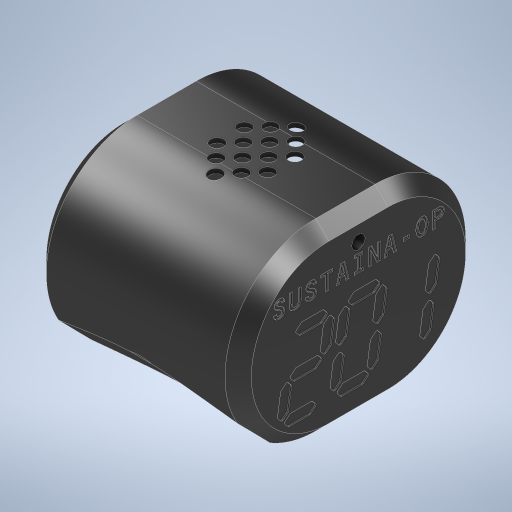
# Autodesk Inventor part: HeadCover
Saved by Autodesk Inventor 2024.2 (Build 282272000, 272)
## iProperties
Created: 2024-06-13
Part Number: HeadCover
Material: ABS Plastic
Document SubType Name: Modeling
Designer: Masato Kubotera
Density: 1.06 g/cm^3
Appearance: Glossy - Black
Author: Masato Kubotera
Autodesk Inventor part; units mm, degrees
(part 1 of 2)
ref_plane "YZ Plane" through (0, 0, 0) normal (1, 0, 0) x (0, 1, 0)
ref_plane "XZ Plane" through (0, 0, 0) normal (0, 1, 0) x (-1, 0, 0)
ref_plane "XY Plane" through (0, 0, 0) normal (0, 0, 1) x (1, 0, 0)
derived "HeadSideFrame_.ipt"
sketch "Sketch1" plane through (0, 0, 0) normal (0, 1, 0) x (-1, 0, 0)
  line L0 (-16.25, -1.5) -> (16.25, -1.5)
  line L1 (-7.25, -1.5) -> (-7.25, 3.5) construction
  line L2 (-7.25, 3.5) -> (7.25, 3.5) construction
  line L3 (0, 3.5) -> (0, -1.5) construction
  line L4 (7.25, -1.5) -> (7.25, 3.5) construction
  line L5 (-13.25, 1) -> (13.25, 1) construction
  line L6 (-7.3, -1.5) -> (-7.3, 3.5)
  line L7 (-7.3, 3.5) -> (7.3, 3.5)
  arc A0 (-4.3, 3.5) -> (-7.3, 3.5) centre (-5.8, 3.5) ccw
  arc A1 (7.3, 3.5) -> (4.3, 3.5) centre (5.8, 3.5) ccw
  line L8 (7.3, -1.5) -> (7.3, 3.5)
  line L9 (-16.25, -1.5) -> (-16.25, 32)
  line L10 (16.25, -1.5) -> (16.25, 65)
  ellipse E0 centre (-16.25, 65) end of major axis (18.25, 65) minor radius 35 (-16.25, 30) -> (-16.25, 100) ccw construction
  line L11 (-16.25, 30) -> (-16.25, 100) construction
  line L12 (-16.25, 65) -> (18.25, 65) construction
  ellipse E1 centre (-16.25, 65) end of major axis (16.25, 65) minor radius 33 (-16.25, 32) -> (16.25, 65) ccw construction
  line L13 (-16.25, 32) -> (-38.75, 32)
  line L14 (-16.25, 98) -> (-38.75, 98)
  line L15 (-27.5, 98) -> (-27.5, 32) construction
  ellipse E2 centre (-38.75, 65) end of major axis (-71.25, 65) minor radius 33 (-38.75, 98) -> (-71.1715, 67.2921) ccw
  ellipse E3 centre (-38.75, 65) end of major axis (-73.25, 65) minor radius 35 (-38.75, 100) -> (-38.75, 30) ccw construction
  line L16 (-38.75, 30) -> (-16.25, 30) construction
  line L17 (-38.75, 100) -> (-16.25, 100) construction
  line L18 (-10.25, 30) -> (10.25, 30)
  line L19 (12.25, 28) -> (12.25, 11)
  line L20 (10.25, 9) -> (-10.25, 9)
  line L21 (-12.25, 11) -> (-12.25, 28)
  line L22 (-12.25, 30) -> (12.25, 9) construction
  line L23 (12.25, 30) -> (-12.25, 9) construction
  arc A2 (-10.25, 30) -> (-12.25, 28) centre (-10.25, 28) ccw
  arc A3 (-12.25, 11) -> (-10.25, 9) centre (-10.25, 11) ccw
  arc A4 (10.25, 9) -> (12.25, 11) centre (10.25, 11) ccw
  arc A5 (12.25, 28) -> (10.25, 30) centre (10.25, 28) ccw
  line L24 (-38.75, 30) -> (-38.75, 100) construction
  line L25 (-38.75, 32) -> (-38.75, 34.8706)
  line L26 (-38.75, 34.8706) -> (-71.1715, 67.2921)
  line L27 (-62.0208, 45.9792) -> (-108, 0) construction
  line L28 (-108, 0) -> (0, 0) construction
  ellipse E4 centre (-38.75, 65) end of major axis (-71.25, 65) minor radius 33 (-71.1715, 67.2921) -> (-38.75, 32) ccw construction
  ellipse E5 centre (-16.25, 65) end of major axis (16.25, 65) minor radius 33 (16.25, 65) -> (-16.25, 98) ccw
  line L29 (-55, 91.5815) -> (0, 91.5815) construction
  line L30 (0, 91.5815) -> (0, 86.5815) construction
  line L31 (0, 86.5815) -> (-55, 86.5815) construction
  line L32 (-55, 86.5815) -> (-55, 91.5815) construction
  line L33 (-55, 91.5815) -> (0, 86.5815) construction
  line L34 (0, 91.5815) -> (-55, 86.5815) construction
  line L35 (-47.5, 91.5815) -> (-47.5, 96.7815) construction
  line L36 (-47.5, 96.7815) -> (-7.5, 96.7815) construction
  line L37 (-7.5, 96.7815) -> (-7.5, 91.5815) construction
  line L38 (-46, 91.5815) -> (-46, 86.5815) construction
  line L39 (-52, 89.0815) -> (-3, 89.0815) construction
  line L40 (-9, 91.5815) -> (-9, 86.5815) construction
  line L41 (-8.95, 86.5315) -> (-46.05, 86.5315)
  line L42 (-46.05, 86.5315) -> (-46.05, 91.6315)
  line L43 (-46.05, 91.6315) -> (-8.95, 91.6315)
  line L44 (-8.95, 91.6315) -> (-8.95, 86.5315)
  line L45 (-8.95, 86.5315) -> (-46.05, 91.6315) construction
  line L46 (-46.05, 86.5315) -> (-8.95, 91.6315) construction
  arc A6 (-43.05, 91.6315) -> (-46.05, 91.6315) centre (-44.55, 91.6315) ccw
  arc A7 (-46.05, 86.5315) -> (-43.05, 86.5315) centre (-44.55, 86.5315) ccw
  arc A8 (-8.95, 91.6315) -> (-11.95, 91.6315) centre (-10.45, 91.6315) ccw
  arc A9 (-11.95, 86.5315) -> (-8.95, 86.5315) centre (-10.45, 86.5315) ccw
  line L47 (-54.1012, 75.112) -> (-60.6066, 68.6066) construction
  line L48 (-60.6066, 68.6066) -> (-39.3934, 47.3934) construction
  line L49 (-39.3934, 47.3934) -> (-32.888, 53.8988) construction
  line L50 (-32.888, 53.8988) -> (-54.1012, 75.112) construction
  line L51 (-56.0104, 64.0104) -> (-72.2739, 47.747) construction
  line L52 (-72.2739, 47.747) -> (-60.253, 35.7261) construction
  line L53 (-60.253, 35.7261) -> (-43.9896, 51.9896) construction
  line L54 (-60.1823, 56.3029) -> (-56.0104, 60.4749) construction
  line L55 (-56.0104, 60.4749) -> (-47.5251, 51.9896) construction
  line L56 (-47.5251, 51.9896) -> (-51.6971, 47.8177) construction
  line L57 (-60.2177, 56.3383) -> (-56.0458, 60.5102)
  line L58 (-56.0458, 60.5102) -> (-47.4898, 51.9542)
  line L59 (-47.4898, 51.9542) -> (-51.6617, 47.7823)
  arc A10 (-47.4898, 51.9542) -> (-49.6111, 54.0756) centre (-48.5504, 53.0149) ccw
  arc A11 (-53.9244, 58.3889) -> (-56.0458, 60.5102) centre (-54.9851, 59.4496) ccw
  line L60 (-62.0208, 62.9497) -> (-45.0503, 45.9792) construction
  line L61 (-51.7678, 56.2322) -> (-55.3033, 52.6967) construction
  line L62 (-59.5459, 56.9393) -> (-51.0607, 48.4541) construction
  circle A12 centre (-45.0503, 45.9792) radius 2.4 construction
  circle A13 centre (-45.0503, 45.9792) radius 1.25 construction
  line L63 (-65.9099, 63.3033) -> (-62.3744, 66.8388) construction
  line L64 (-44.6967, 42.0901) -> (-41.1612, 45.6256) construction
  line L65 (-29.75, 40.55) -> (7.25, 40.55) construction
  line L66 (7.25, 40.55) -> (7.25, 35.55) construction
  line L67 (7.25, 35.55) -> (-29.75, 35.55) construction
  line L68 (-29.75, 35.55) -> (-29.75, 40.55) construction
  line L69 (-29.75, 40.55) -> (7.25, 35.55) construction
  line L70 (7.25, 40.55) -> (-29.75, 35.55) construction
  line L71 (-35.75, 38.05) -> (13.25, 38.05) construction
  line L72 (-11.25, 40.55) -> (-11.25, 35.55) construction
  line L73 (-38.75, 40.55) -> (-38.75, 35.55) construction
  line L74 (16.25, 40.55) -> (16.25, 35.55) construction
  line L75 (-29.8, 40.6) -> (7.3, 40.6)
  line L76 (7.3, 40.6) -> (7.3, 35.5)
  line L77 (7.3, 35.5) -> (-29.8, 35.5)
  line L78 (-29.8, 35.5) -> (-29.8, 40.6)
  line L79 (-29.8, 40.6) -> (7.3, 35.5) construction
  line L80 (7.3, 40.6) -> (-29.8, 35.5) construction
  arc A14 (4.3, 35.5) -> (7.3, 35.5) centre (5.8, 35.5) ccw
  arc A15 (7.3, 40.6) -> (4.3, 40.6) centre (5.8, 40.6) ccw
  arc A16 (-26.8, 40.6) -> (-29.8, 40.6) centre (-28.3, 40.6) ccw
  arc A17 (-29.8, 35.5) -> (-26.8, 35.5) centre (-28.3, 35.5) ccw
  line L81 (-59.7893, 83.0315) -> (4.7893, 83.0315)
  line L82 (-63.4241, 77.3638) -> (-30.1603, 44.1)
  ellipse E6 centre (-16.25, 65) end of major axis (11.25, 65) minor radius 28.0012 (2.0513, 44.1) -> (11.25, 65) ccw
  ellipse E7 centre (-16.25, 65) end of major axis (11.25, 65) minor radius 28.0012 (11.25, 65) -> (4.7893, 83.0315) ccw
  ellipse E8 centre (-38.75, 65) end of major axis (-66.25, 65) minor radius 28.0012 (-59.7893, 83.0315) -> (-63.4241, 77.3638) ccw
  line L83 (-16.25, 65) -> (8.5857, 86.2852) construction
  line L84 (-30.1603, 44.1) -> (2.0513, 44.1)
  line L85 (-62.0208, 45.9792) -> (-32.844, 9.9488)
  line L86 (-32.844, 9.9488) -> (-98.0512, 75.156)
  line L87 (-98.0512, 75.156) -> (-62.0208, 45.9792)
  line L88 (-38.75, 65) -> (-73.25, 65) construction
  point P0 (0, 1)
  point P1 (0, 19.5)
  point P2 (5.8, 5)
  point P3 (-27.5, 89.0815)
  point P4 (-53.5355, 54.4645)
  point P5 (-50, 58)
  point P6 (-11.25, 38.05)
  point P7 (-11.25, 38.05)
  point P8 (-10.45, 85.0315)
  point P9 (-28.3, 34)
  point P10 (5.8, 42.1)
  point P11 (-27.5, 89.0815)
sketch "Sketch2" plane through (0, 0, 0) normal (0, 1, 0) x (-1, 0, 0)
  ellipse E0 centre (-38.75, 65) end of major axis (-38.75, 30) minor radius 34.5 (-38.75, 100) -> (-38.75, 30) ccw projected
  line L0 (-38.75, 100) -> (-16.25, 100) projected
  ellipse E1 centre (-16.25, 65) end of major axis (-16.25, 100) minor radius 34.5 (-16.25, 30) -> (-16.25, 100) ccw projected
  line L1 (-38.75, 30) -> (-16.25, 30) projected
  line L2 (-62.0208, 45.9792) -> (-32.844, 9.9488) projected
  line L3 (-32.844, 9.9488) -> (-98.0512, 75.156) projected
  line L4 (-98.0512, 75.156) -> (-62.0208, 45.9792) projected
  ellipse E2 centre (-38.75, 65) end of major axis (-38.75, 98.25) minor radius 32.75 (-38.75, 98.25) -> (-71.5, 65) ccw
  line L5 (-38.75, 30) -> (-38.75, 100) construction
  ellipse E3 centre (-38.75, 65) end of major axis (-38.75, 32) minor radius 32.5 (-38.75, 98) -> (-71.1715, 67.2921) ccw projected
  line L6 (-38.75, 65) -> (-73.25, 65) construction
  ellipse E4 centre (-38.75, 65) end of major axis (-38.75, 32) minor radius 32.5 (-71.1715, 67.2921) -> (-38.75, 32) ccw construction
  ellipse E5 centre (-38.75, 65) end of major axis (-38.75, 98.25) minor radius 32.75 (-71.5, 65) -> (-38.75, 31.75) ccw
  line L7 (-27.5, 98) -> (-27.5, 32) construction
  ellipse E6 centre (-16.25, 65) end of major axis (-16.25, 98.25) minor radius 32.75 (6.7317, 88.6887) -> (-16.25, 98.25) ccw
  line L8 (-38.75, 98.25) -> (-16.25, 98.25)
  line L9 (6.7317, 88.6887) -> (14.4481, 80.9723) construction
  line L10 (-38.75, 34.8706) -> (-71.1715, 67.2921) projected
  line L11 (-38.75, 32) -> (-38.75, 34.8706) projected
  line L12 (-39, 34.7671) -> (-39, 30.0009)
  line L13 (-39, 34.7671) -> (-71.4285, 67.1956)
  line L14 (-62.0208, 45.9792) -> (-108, 0) projected
  line L15 (-74.2864, 51.3912) -> (-64.9553, 60.7224)
  line L16 (-65.4476, 42.5524) -> (-56.1165, 51.8835)
  arc A0 (6.7317, 88.6887) -> (7.9691, 89.9261) centre (7.3504, 89.3074) ccw
  point P0 (0, 0)
  point P1 (-71.25, 65)
  point P2 (-66.4476, 43.5524)
  point P3 (-71.7886, 53.889)
  point P4 (-39, 31.751)
  point P5 (-70.1445, 55.5331)
  point P6 (-71.5449, 54.1328)
  point P7 (-27.5, 89.0815)
  dimension "d1" = 0.25
  dimension "d4" = 0.25
  dimension "d5" = 0.25
  dimension "d41" = 25
  dimension "d52" = 0.25
  constraints: 12 end point, 9 point on line, 3 vertical, 2 horizontal, 2 parallel, 2 point on circle, 2 symmetric about line, 1 centre point, 1 coincident, 1 midpoint, 1 perpendicular, 25 other
  measures "d1" distance of L8.start point (-38.75, 98)
  measures "d4" distance of point (-71.5, 65) point (-71.25, 65)
  measures "d5" distance between parallel lines of L13 L10
  measures "d41" diameter of L15 L16
  measures "d52" distance between parallel lines of L5 L12
extrude "Extrusion1" add sketch "Sketch2" along normal blind 39 contours L12 L13 E2 L8 E6 A0 E1 L1 E0 | E0 L2 E5 L12 | E0 L14 E5 L2 | E5 L2 L16 L13 L12 | E5 L14 L2 | A0 E6 L8 E2 E5 L15 E0 L0 E1 | E0 L4 E5 L14 | L14 E5 L4 | L4 E5 L15 L13 L16 | E0 L15 E5 L4 | L15 E5 E2 L13
chamfer "C5" distance 5 angle 45 4 edges at (73.25, 39, 65) (27.5, 39, 30) (-18.25, 39, 65) (27.5, 39, 100)
revolve "Revolution1" cut sketch "Sketch2" angle 180 about axis through (62.0208, 0, 45.9792) along (-0.7071068, 0, 0.7071068) contours L14 L3 L15 L4 E0 | E0 L4 E5 L14 | L14 E5 L4 | L4 E5 L15 L13 L16 | L4 L15 E0 | E0 L15 E5 L4 | L3 L4 L15
extrude "Extrusion2" cut sketch "Sketch2" along normal blind 33 contours L12 L13 E2 L8 E6 A0 E1 L1 E0
sketch "Sketch4" plane through (16.25, 0, 100) normal (0, 0, 1) x (1, 0, 0)
  line L0 (-8.75, -14.15) -> (31.25, -14.15) construction
  line L1 (31.25, -14.15) -> (31.25, 14.15) construction
  line L2 (31.25, 14.15) -> (-8.75, 14.15) construction
  line L3 (-8.75, 14.15) -> (-8.75, -14.15) construction
  line L4 (0, 0) -> (22.5, 0) projected
  line L5 (-8.75, -14.15) -> (31.25, 14.15) construction
  line L6 (31.25, -14.15) -> (-8.75, 14.15) construction
  line L7 (57, 0) -> (22.5, 0) projected
  arc A0 (17.1, -12.15) -> (17.1, 12.15) centre (17.1, 0) ccw
  line L8 (17.1, 12.15) -> (5.4, 12.15)
  line L9 (11.25, 14.15) -> (11.25, -14.15) construction
  arc A1 (5.4, 12.15) -> (5.4, -12.15) centre (5.4, 0) ccw
  line L10 (17.1, -12.15) -> (5.4, -12.15)
  line L11 (0, 0) -> (-24.2191, 0) projected
  circle A2 centre (-4.25, 0) radius 2.5
  circle A3 centre (0.9167, 4.8129) radius 2.5
  circle A4 centre (6.0833, 9.6258) radius 2.5
  circle A5 centre (6.0833, 0) radius 2.5
  circle A6 centre (11.25, 4.8129) radius 2.5
  line L12 (6.0833, 0) -> (6.0833, 9.6258) construction
  line L13 (0.9167, 4.8129) -> (11.25, 4.8129) construction
  line L14 (0.9167, 4.8129) -> (0.9167, 0) construction
  circle A7 centre (26.75, 0) radius 2.5
  circle A8 centre (21.5833, 4.8129) radius 2.5
  circle A9 centre (16.4167, 9.6258) radius 2.5
  circle A10 centre (16.4167, 0) radius 2.5
  point P0 (-16.25, 0)
  point P1 (11.25, 0)
  point P2 (55.2949, 0)
  point P3 (29.25, 0)
  point P4 (31.25, 0)
  point P5 (5.4, -12.15)
  point P6 (6.0833, 4.8129)
  dimension "d44" = 40
  dimension "d45" = 28.3
  dimension "d50" = 2
  dimension "d51" = 2
  dimension "d64" = 5
  constraints: 24 end point, 11 centre point, 9 symmetric about line, 8 midpoint, 5 point on circle, 5 point on line, 4 equal radius, 3 horizontal, 3 tangent, 2 parallel, 2 vertical, 1 perpendicular, 6 other
  measures "d44" distance of L2.end L1.end
  measures "d45" distance of L1.end L0.end
  measures "d50" distance of point (29.25, 0) point (31.25, 0)
  measures "d51" distance from line of L2 L8.start
  measures "d64" diameter of A2
extrude "Extrusion3" cut sketch "Sketch4" against normal blind 5 contours A10 L4 | L4 A10 | A7 L7 | L7 A7 | A5 L4 | L4 A5 | A2 L11 | L11 A2 | A3 | A4 | A6 | A8 | A9
fillet "R2" radius 2 2 edges at (39, 16.5, 34.7671) (71.4285, 16.5, 67.1956)
mirror "Mirror1" about plane through (0, 0, 0) normal (0, 1, 0)
sketch "Sketch3" plane through (0, 39, 0) normal (0, 1, 0) x (1, 0, 0)
  line L0 (16.25, -35) -> (38.75, -35) projected
  line L1 (38.75, -95) -> (16.25, -95) projected
  line L2 (23.91, -55.4167) -> (31.6756, -55.4167)
  line L3 (27.7928, -55.4167) -> (27.2072, -59.5833) construction
  line L4 (23.3244, -59.5833) -> (31.09, -59.5833)
  line L5 (21.6569, -57.9744) -> (22.85, -59.3653)
  arc A0 (21.7244, -57.0931) -> (21.6569, -57.9744) centre (22.1313, -57.5675) ccw
  line L6 (20.7082, -58.7882) -> (21.9013, -60.1791)
  arc A1 (22.0446, -60.6812) -> (21.9013, -60.1791) centre (21.4269, -60.586) ccw
  arc A2 (22.85, -59.3653) -> (23.3244, -59.5833) centre (23.3244, -58.9583) ccw
  arc A3 (36.9518, -54.7534) -> (37.1626, -54.3742) centre (36.5449, -54.2791) ccw
  line L7 (36.9518, -54.7534) -> (35.1731, -56.2792)
  arc A4 (34.2918, -56.2118) -> (35.1731, -56.2792) centre (34.7662, -55.8048) ccw
  line L8 (38.3444, -46.699) -> (37.1626, -54.3742)
  arc A5 (34.8551, -58.7882) -> (33.9738, -58.7208) centre (34.3807, -59.1952) ccw
  line L9 (34.8551, -58.7882) -> (36.0482, -60.1791)
  arc A6 (36.1915, -60.6812) -> (36.0482, -60.1791) centre (35.5738, -60.586) ccw
  arc A7 (22.8049, -54.7534) -> (23.0157, -54.3742) centre (22.398, -54.2791) ccw
  line L10 (23.5031, -55.5673) -> (21.7244, -57.0931)
  line L11 (22.8049, -54.7534) -> (21.0262, -56.2792)
  arc A8 (20.1449, -56.2118) -> (21.0262, -56.2792) centre (20.6193, -55.8048) ccw
  line L12 (19.9903, -46.6437) -> (18.8085, -54.3188)
  line L13 (24.1975, -46.699) -> (23.0157, -54.3742)
  line L14 (34.1372, -46.6437) -> (32.9554, -54.3188)
  arc A9 (38.3444, -46.699) -> (38.2011, -46.197) centre (37.7267, -46.6039) ccw
  arc A10 (18.8085, -54.3188) -> (18.9518, -54.8209) centre (19.4262, -54.414) ccw
  arc A11 (32.1951, -60.2466) -> (31.9843, -60.6258) centre (32.602, -60.7209) ccw
  line L15 (31.4969, -59.4327) -> (33.2756, -57.9069)
  arc A12 (33.2756, -57.9069) -> (33.3431, -57.0256) centre (32.8687, -57.4325) ccw
  arc A13 (32.9554, -54.3188) -> (33.0987, -54.8209) centre (33.5731, -54.414) ccw
  line L16 (34.2918, -56.2118) -> (33.0987, -54.8209)
  arc A14 (20.2011, -46.2645) -> (19.9903, -46.6437) centre (20.608, -46.7388) ccw
  line L17 (25.4773, -45.6012) -> (33.2429, -45.6012)
  arc A15 (34.3479, -46.2645) -> (34.1372, -46.6437) centre (34.7549, -46.7388) ccw
  arc A16 (23.91, -55.4167) -> (23.5031, -55.5673) centre (23.91, -56.0417) ccw
  arc A17 (24.1975, -46.699) -> (24.0542, -46.197) centre (23.5798, -46.6039) ccw
  arc A18 (18.0482, -60.2466) -> (17.8374, -60.6258) centre (18.4551, -60.7209) ccw
  arc A19 (25.0029, -45.3831) -> (25.4773, -45.6012) centre (25.4773, -44.9762) ccw
  line L18 (22.8611, -44.8061) -> (24.0542, -46.197)
  line L19 (36.1266, -44.7387) -> (34.3479, -46.2645)
  line L20 (22.4541, -44.3317) -> (20.5519, -56.6861) construction
  line L21 (23.8098, -43.9923) -> (25.0029, -45.3831)
  line L22 (35.9029, -43.5179) -> (23.4029, -43.5179) construction
  line L23 (25.656, -41.5852) -> (23.8773, -43.111)
  line L24 (26.0629, -41.4346) -> (33.8285, -41.4346)
  arc A20 (23.8773, -43.111) -> (23.8098, -43.9923) centre (24.2842, -43.5853) ccw
  arc A21 (26.0629, -41.4346) -> (25.656, -41.5852) centre (26.0629, -42.0596) ccw
  line L25 (21.9798, -44.7387) -> (20.2011, -46.2645)
  line L26 (17.8374, -60.6258) -> (16.6556, -68.301)
  line L27 (20.1449, -56.2118) -> (18.9518, -54.8209)
  arc A22 (22.8611, -44.8061) -> (21.9798, -44.7387) centre (22.3867, -45.213) ccw
  line L28 (22.0446, -60.6812) -> (20.8628, -68.3563)
  arc A23 (21.7571, -69.3988) -> (21.3502, -69.5494) centre (21.7571, -70.0238) ccw
  arc A24 (31.09, -59.5833) -> (31.4969, -59.4327) centre (31.09, -58.9583) ccw
  line L29 (33.9738, -58.7208) -> (32.1951, -60.2466)
  line L30 (21.7571, -69.3988) -> (29.5227, -69.3988)
  arc A25 (30.8025, -68.301) -> (30.9458, -68.803) centre (31.4202, -68.3961) ccw
  line L31 (31.9843, -60.6258) -> (30.8025, -68.301)
  line L32 (32.1389, -70.1939) -> (30.9458, -68.803)
  arc A26 (32.1389, -70.1939) -> (33.0202, -70.2613) centre (32.6133, -69.787) ccw
  arc A27 (19.5715, -71.0752) -> (19.504, -71.9565) centre (19.9784, -71.5496) ccw
  line L33 (19.504, -71.9565) -> (20.6971, -73.3474)
  line L34 (21.1715, -73.5654) -> (28.9371, -73.5654)
  line L35 (20.6521, -68.7355) -> (18.8734, -70.2613)
  arc A28 (17.992, -70.1939) -> (18.8734, -70.2613) centre (18.4664, -69.787) ccw
  line L36 (17.992, -70.1939) -> (16.7989, -68.803)
  arc A29 (28.9371, -73.5654) -> (29.344, -73.4148) centre (28.9371, -72.9404) ccw
  arc A30 (29.9971, -69.6169) -> (29.5227, -69.3988) centre (29.5227, -70.0238) ccw
  line L37 (29.344, -73.4148) -> (31.1227, -71.889)
  arc A31 (31.1227, -71.889) -> (31.1902, -71.0077) centre (30.7158, -71.4147) ccw
  line L38 (29.9971, -69.6169) -> (31.1902, -71.0077)
  arc A32 (20.6971, -73.3474) -> (21.1715, -73.5654) centre (21.1715, -72.9404) ccw
  arc A33 (20.7082, -58.7882) -> (19.8269, -58.7208) centre (20.2338, -59.1952) ccw
  line L39 (19.8269, -58.7208) -> (18.0482, -60.2466)
  arc A34 (20.6521, -68.7355) -> (20.8628, -68.3563) centre (20.2451, -68.2612) ccw
  arc A35 (16.6556, -68.301) -> (16.7989, -68.803) centre (17.2733, -68.3961) ccw
  line L40 (21.3502, -69.5494) -> (19.5715, -71.0752)
  arc A36 (32.15, -55.6347) -> (31.6756, -55.4167) centre (31.6756, -56.0417) ccw
  line L41 (33.6498, -45.4506) -> (35.4285, -43.9248)
  line L42 (37.008, -44.8061) -> (38.2011, -46.197)
  arc A37 (37.008, -44.8061) -> (36.1266, -44.7387) centre (36.5336, -45.213) ccw
  arc A38 (35.4285, -43.9248) -> (35.496, -43.0435) centre (35.0216, -43.4504) ccw
  arc A39 (34.3029, -41.6526) -> (33.8285, -41.4346) centre (33.8285, -42.0596) ccw
  line L43 (36.1915, -60.6812) -> (35.0097, -68.3563)
  line L44 (34.7989, -68.7355) -> (33.0202, -70.2613)
  arc A40 (33.2429, -45.6012) -> (33.6498, -45.4506) centre (33.2429, -44.9762) ccw
  line L45 (34.3029, -41.6526) -> (35.496, -43.0435)
  line L46 (32.15, -55.6347) -> (33.3431, -57.0256)
  arc A41 (34.7989, -68.7355) -> (35.0097, -68.3563) centre (34.392, -68.2612) ccw
  line L47 (7.7928, -55.4167) -> (7.2072, -59.5833) construction
  line L48 (3.91, -55.4167) -> (11.6756, -55.4167)
  line L49 (3.3244, -59.5833) -> (11.09, -59.5833)
  arc A42 (5.0029, -45.3831) -> (5.4773, -45.6012) centre (5.4773, -44.9762) ccw
  line L50 (14.1372, -46.6437) -> (12.9554, -54.3188)
  arc A43 (14.3479, -46.2645) -> (14.1372, -46.6437) centre (14.7549, -46.7388) ccw
  line L51 (18.3444, -46.699) -> (17.1626, -54.3742)
  line L52 (5.4773, -45.6012) -> (13.2429, -45.6012)
  line L53 (16.1266, -44.7387) -> (14.3479, -46.2645)
  arc A44 (16.9518, -54.7534) -> (17.1626, -54.3742) centre (16.5449, -54.2791) ccw
  line L54 (16.9518, -54.7534) -> (15.1731, -56.2792)
  arc A45 (14.2918, -56.2118) -> (15.1731, -56.2792) centre (14.7662, -55.8048) ccw
  arc A46 (14.8551, -58.7882) -> (13.9738, -58.7208) centre (14.3807, -59.1952) ccw
  line L55 (14.8551, -58.7882) -> (16.0482, -60.1791)
  line L56 (1.6569, -57.9744) -> (2.85, -59.3653)
  line L57 (0.7082, -58.7882) -> (1.9013, -60.1791)
  arc A47 (2.0446, -60.6812) -> (1.9013, -60.1791) centre (1.4269, -60.586) ccw
  arc A48 (2.85, -59.3653) -> (3.3244, -59.5833) centre (3.3244, -58.9583) ccw
  arc A49 (0.7082, -58.7882) -> (-0.1731, -58.7208) centre (0.2338, -59.1952) ccw
  line L58 (-0.1731, -58.7208) -> (-1.9518, -60.2466)
  arc A50 (-1.9518, -60.2466) -> (-2.1626, -60.6258) centre (-1.5449, -60.7209) ccw
  line L59 (-2.1626, -60.6258) -> (-3.3444, -68.301)
  line L60 (2.0446, -60.6812) -> (0.8628, -68.3563)
  line L61 (3.8098, -43.9923) -> (5.0029, -45.3831)
  arc A51 (4.1975, -46.699) -> (4.0542, -46.197) centre (3.5798, -46.6039) ccw
  line L62 (2.8611, -44.8061) -> (4.0542, -46.197)
  line L63 (1.9798, -44.7387) -> (0.2011, -46.2645)
  line L64 (4.1975, -46.699) -> (3.0157, -54.3742)
  arc A52 (0.2011, -46.2645) -> (-0.0097, -46.6437) centre (0.608, -46.7388) ccw
  arc A53 (3.91, -55.4167) -> (3.5031, -55.5673) centre (3.91, -56.0417) ccw
  arc A54 (2.8049, -54.7534) -> (3.0157, -54.3742) centre (2.398, -54.2791) ccw
  line L65 (2.4541, -44.3317) -> (0.5519, -56.6861) construction
  line L66 (-0.0097, -46.6437) -> (-1.1915, -54.3188)
  arc A55 (1.7244, -57.0931) -> (1.6569, -57.9744) centre (2.1313, -57.5675) ccw
  line L67 (2.8049, -54.7534) -> (1.0262, -56.2792)
  line L68 (3.5031, -55.5673) -> (1.7244, -57.0931)
  arc A56 (0.1449, -56.2118) -> (1.0262, -56.2792) centre (0.6193, -55.8048) ccw
  arc A57 (12.15, -55.6347) -> (11.6756, -55.4167) centre (11.6756, -56.0417) ccw
  arc A58 (12.9554, -54.3188) -> (13.0987, -54.8209) centre (13.5731, -54.414) ccw
  line L69 (14.2918, -56.2118) -> (13.0987, -54.8209)
  line L70 (12.15, -55.6347) -> (13.3431, -57.0256)
  line L71 (11.4969, -59.4327) -> (13.2756, -57.9069)
  arc A59 (13.2756, -57.9069) -> (13.3431, -57.0256) centre (12.8687, -57.4325) ccw
  arc A60 (-1.1915, -54.3188) -> (-1.0482, -54.8209) centre (-0.5738, -54.414) ccw
  line L72 (0.1449, -56.2118) -> (-1.0482, -54.8209)
  arc A61 (10.8025, -68.301) -> (10.9458, -68.803) centre (11.4202, -68.3961) ccw
  arc A62 (11.09, -59.5833) -> (11.4969, -59.4327) centre (11.09, -58.9583) ccw
  line L73 (11.9843, -60.6258) -> (10.8025, -68.301)
  arc A63 (12.1951, -60.2466) -> (11.9843, -60.6258) centre (12.602, -60.7209) ccw
  line L74 (12.1389, -70.1939) -> (10.9458, -68.803)
  line L75 (14.7989, -68.7355) -> (13.0202, -70.2613)
  line L76 (16.1915, -60.6812) -> (15.0097, -68.3563)
  line L77 (13.9738, -58.7208) -> (12.1951, -60.2466)
  arc A64 (16.1915, -60.6812) -> (16.0482, -60.1791) centre (15.5738, -60.586) ccw
  arc A65 (18.3444, -46.699) -> (18.2011, -46.197) centre (17.7267, -46.6039) ccw
  arc A66 (14.3029, -41.6526) -> (13.8285, -41.4346) centre (13.8285, -42.0596) ccw
  line L78 (14.3029, -41.6526) -> (15.496, -43.0435)
  arc A67 (15.4285, -43.9248) -> (15.496, -43.0435) centre (15.0216, -43.4504) ccw
  line L79 (13.6498, -45.4506) -> (15.4285, -43.9248)
  arc A68 (17.008, -44.8061) -> (16.1266, -44.7387) centre (16.5336, -45.213) ccw
  line L80 (17.008, -44.8061) -> (18.2011, -46.197)
  arc A69 (13.2429, -45.6012) -> (13.6498, -45.4506) centre (13.2429, -44.9762) ccw
  arc A70 (1.7571, -69.3988) -> (1.3502, -69.5494) centre (1.7571, -70.0238) ccw
  line L81 (1.7571, -69.3988) -> (9.5227, -69.3988)
  arc A71 (8.9371, -73.5654) -> (9.344, -73.4148) centre (8.9371, -72.9404) ccw
  arc A72 (9.9971, -69.6169) -> (9.5227, -69.3988) centre (9.5227, -70.0238) ccw
  line L82 (9.344, -73.4148) -> (11.1227, -71.889)
  line L83 (9.9971, -69.6169) -> (11.1902, -71.0077)
  arc A73 (11.1227, -71.889) -> (11.1902, -71.0077) centre (10.7158, -71.4147) ccw
  arc A74 (12.1389, -70.1939) -> (13.0202, -70.2613) centre (12.6133, -69.787) ccw
  line L84 (1.1715, -73.5654) -> (8.9371, -73.5654)
  arc A75 (-0.4285, -71.0752) -> (-0.496, -71.9565) centre (-0.0216, -71.5496) ccw
  line L85 (-0.496, -71.9565) -> (0.6971, -73.3474)
  arc A76 (14.7989, -68.7355) -> (15.0097, -68.3563) centre (14.392, -68.2612) ccw
  arc A77 (0.6971, -73.3474) -> (1.1715, -73.5654) centre (1.1715, -72.9404) ccw
  arc A78 (0.6521, -68.7355) -> (0.8628, -68.3563) centre (0.2451, -68.2612) ccw
  line L86 (1.3502, -69.5494) -> (-0.4285, -71.0752)
  line L87 (0.6521, -68.7355) -> (-1.1266, -70.2613)
  arc A79 (-2.008, -70.1939) -> (-1.1266, -70.2613) centre (-1.5336, -69.787) ccw
  line L88 (-2.008, -70.1939) -> (-3.2011, -68.803)
  arc A80 (-3.3444, -68.301) -> (-3.2011, -68.803) centre (-2.7267, -68.3961) ccw
  line L89 (15.9029, -43.5179) -> (3.4029, -43.5179) construction
  line L90 (6.0629, -41.4346) -> (13.8285, -41.4346)
  arc A81 (6.0629, -41.4346) -> (5.656, -41.5852) centre (6.0629, -42.0596) ccw
  line L91 (5.656, -41.5852) -> (3.8773, -43.111)
  arc A82 (3.8773, -43.111) -> (3.8098, -43.9923) centre (4.2842, -43.5853) ccw
  arc A83 (2.8611, -44.8061) -> (1.9798, -44.7387) centre (2.3867, -45.213) ccw
  line L92 (47.7928, -55.4167) -> (47.2072, -59.5833) construction
  line L93 (43.91, -55.4167) -> (51.6756, -55.4167)
  line L94 (43.3244, -59.5833) -> (51.09, -59.5833)
  arc A84 (45.0029, -45.3831) -> (45.4773, -45.6012) centre (45.4773, -44.9762) ccw
  line L95 (54.1372, -46.6437) -> (52.9554, -54.3188)
  arc A85 (54.3479, -46.2645) -> (54.1372, -46.6437) centre (54.7549, -46.7388) ccw
  line L96 (58.3444, -46.699) -> (57.1626, -54.3742)
  line L97 (45.4773, -45.6012) -> (53.2429, -45.6012)
  line L98 (56.1266, -44.7387) -> (54.3479, -46.2645)
  arc A86 (56.9518, -54.7534) -> (57.1626, -54.3742) centre (56.5449, -54.2791) ccw
  line L99 (56.9518, -54.7534) -> (55.1731, -56.2792)
  arc A87 (54.2918, -56.2118) -> (55.1731, -56.2792) centre (54.7662, -55.8048) ccw
  arc A88 (54.8551, -58.7882) -> (53.9738, -58.7208) centre (54.3807, -59.1952) ccw
  line L100 (54.8551, -58.7882) -> (56.0482, -60.1791)
  line L101 (41.6569, -57.9744) -> (42.85, -59.3653)
  line L102 (40.7082, -58.7882) -> (41.9013, -60.1791)
  arc A89 (42.0446, -60.6812) -> (41.9013, -60.1791) centre (41.4269, -60.586) ccw
  arc A90 (42.85, -59.3653) -> (43.3244, -59.5833) centre (43.3244, -58.9583) ccw
  arc A91 (40.7082, -58.7882) -> (39.8269, -58.7208) centre (40.2338, -59.1952) ccw
  line L103 (39.8269, -58.7208) -> (38.0482, -60.2466)
  arc A92 (38.0482, -60.2466) -> (37.8374, -60.6258) centre (38.4551, -60.7209) ccw
  line L104 (37.8374, -60.6258) -> (36.6556, -68.301)
  line L105 (42.0446, -60.6812) -> (40.8628, -68.3563)
  line L106 (43.8098, -43.9923) -> (45.0029, -45.3831)
  arc A93 (44.1975, -46.699) -> (44.0542, -46.197) centre (43.5798, -46.6039) ccw
  line L107 (42.8611, -44.8061) -> (44.0542, -46.197)
  line L108 (41.9798, -44.7387) -> (40.2011, -46.2645)
  line L109 (44.1975, -46.699) -> (43.0157, -54.3742)
  arc A94 (40.2011, -46.2645) -> (39.9903, -46.6437) centre (40.608, -46.7388) ccw
  arc A95 (43.91, -55.4167) -> (43.5031, -55.5673) centre (43.91, -56.0417) ccw
  arc A96 (42.8049, -54.7534) -> (43.0157, -54.3742) centre (42.398, -54.2791) ccw
  line L110 (42.4541, -44.3317) -> (40.5519, -56.6861) construction
  line L111 (39.9903, -46.6437) -> (38.8085, -54.3188)
  arc A97 (41.7244, -57.0931) -> (41.6569, -57.9744) centre (42.1313, -57.5675) ccw
  line L112 (42.8049, -54.7534) -> (41.0262, -56.2792)
  line L113 (43.5031, -55.5673) -> (41.7244, -57.0931)
  arc A98 (40.1449, -56.2118) -> (41.0262, -56.2792) centre (40.6193, -55.8048) ccw
  arc A99 (52.15, -55.6347) -> (51.6756, -55.4167) centre (51.6756, -56.0417) ccw
  arc A100 (52.9554, -54.3188) -> (53.0987, -54.8209) centre (53.5731, -54.414) ccw
  line L114 (54.2918, -56.2118) -> (53.0987, -54.8209)
  line L115 (52.15, -55.6347) -> (53.3431, -57.0256)
  line L116 (51.4969, -59.4327) -> (53.2756, -57.9069)
  arc A101 (53.2756, -57.9069) -> (53.3431, -57.0256) centre (52.8687, -57.4325) ccw
  arc A102 (38.8085, -54.3188) -> (38.9518, -54.8209) centre (39.4262, -54.414) ccw
  line L117 (40.1449, -56.2118) -> (38.9518, -54.8209)
  arc A103 (50.8025, -68.301) -> (50.9458, -68.803) centre (51.4202, -68.3961) ccw
  arc A104 (51.09, -59.5833) -> (51.4969, -59.4327) centre (51.09, -58.9583) ccw
  line L118 (51.9843, -60.6258) -> (50.8025, -68.301)
  arc A105 (52.1951, -60.2466) -> (51.9843, -60.6258) centre (52.602, -60.7209) ccw
  line L119 (52.1389, -70.1939) -> (50.9458, -68.803)
  line L120 (54.7989, -68.7355) -> (53.0202, -70.2613)
  line L121 (56.1915, -60.6812) -> (55.0097, -68.3563)
  line L122 (53.9738, -58.7208) -> (52.1951, -60.2466)
  arc A106 (56.1915, -60.6812) -> (56.0482, -60.1791) centre (55.5738, -60.586) ccw
  arc A107 (58.3444, -46.699) -> (58.2011, -46.197) centre (57.7267, -46.6039) ccw
  arc A108 (54.3029, -41.6526) -> (53.8285, -41.4346) centre (53.8285, -42.0596) ccw
  line L123 (54.3029, -41.6526) -> (55.496, -43.0435)
  arc A109 (55.4285, -43.9248) -> (55.496, -43.0435) centre (55.0216, -43.4504) ccw
  line L124 (53.6498, -45.4506) -> (55.4285, -43.9248)
  arc A110 (57.008, -44.8061) -> (56.1266, -44.7387) centre (56.5336, -45.213) ccw
  line L125 (57.008, -44.8061) -> (58.2011, -46.197)
  arc A111 (53.2429, -45.6012) -> (53.6498, -45.4506) centre (53.2429, -44.9762) ccw
  arc A112 (41.7571, -69.3988) -> (41.3502, -69.5494) centre (41.7571, -70.0238) ccw
  line L126 (41.7571, -69.3988) -> (49.5227, -69.3988)
  arc A113 (48.9371, -73.5654) -> (49.344, -73.4148) centre (48.9371, -72.9404) ccw
  arc A114 (49.9971, -69.6169) -> (49.5227, -69.3988) centre (49.5227, -70.0238) ccw
  line L127 (49.344, -73.4148) -> (51.1227, -71.889)
  line L128 (49.9971, -69.6169) -> (51.1902, -71.0077)
  arc A115 (51.1227, -71.889) -> (51.1902, -71.0077) centre (50.7158, -71.4147) ccw
  arc A116 (52.1389, -70.1939) -> (53.0202, -70.2613) centre (52.6133, -69.787) ccw
  line L129 (41.1715, -73.5654) -> (48.9371, -73.5654)
  arc A117 (39.5715, -71.0752) -> (39.504, -71.9565) centre (39.9784, -71.5496) ccw
  line L130 (39.504, -71.9565) -> (40.6971, -73.3474)
  arc A118 (54.7989, -68.7355) -> (55.0097, -68.3563) centre (54.392, -68.2612) ccw
  arc A119 (40.6971, -73.3474) -> (41.1715, -73.5654) centre (41.1715, -72.9404) ccw
  arc A120 (40.6521, -68.7355) -> (40.8628, -68.3563) centre (40.2451, -68.2612) ccw
  line L131 (41.3502, -69.5494) -> (39.5715, -71.0752)
  line L132 (40.6521, -68.7355) -> (38.8734, -70.2613)
  arc A121 (37.992, -70.1939) -> (38.8734, -70.2613) centre (38.4664, -69.787) ccw
  line L133 (37.992, -70.1939) -> (36.7989, -68.803)
  arc A122 (36.6556, -68.301) -> (36.7989, -68.803) centre (37.2733, -68.3961) ccw
  line L134 (55.9029, -43.5179) -> (43.4029, -43.5179) construction
  line L135 (46.0629, -41.4346) -> (53.8285, -41.4346)
  arc A123 (46.0629, -41.4346) -> (45.656, -41.5852) centre (46.0629, -42.0596) ccw
  line L136 (45.656, -41.5852) -> (43.8773, -43.111)
  arc A124 (43.8773, -43.111) -> (43.8098, -43.9923) centre (44.2842, -43.5853) ccw
  arc A125 (42.8611, -44.8061) -> (41.9798, -44.7387) centre (42.3867, -45.213) ccw
  line L137 (27.7928, -55.4167) -> (27.2072, -59.5833) construction
  line L138 (23.91, -55.4167) -> (31.6756, -55.4167)
  line L139 (23.3244, -59.5833) -> (31.09, -59.5833)
  arc A126 (25.0029, -45.3831) -> (25.4773, -45.6012) centre (25.4773, -44.9762) ccw
  line L140 (34.1372, -46.6437) -> (32.9554, -54.3188)
  arc A127 (34.3479, -46.2645) -> (34.1372, -46.6437) centre (34.7549, -46.7388) ccw
  line L141 (38.3444, -46.699) -> (37.1626, -54.3742)
  line L142 (25.4773, -45.6012) -> (33.2429, -45.6012)
  line L143 (36.1266, -44.7387) -> (34.3479, -46.2645)
  arc A128 (36.9518, -54.7534) -> (37.1626, -54.3742) centre (36.5449, -54.2791) ccw
  line L144 (36.9518, -54.7534) -> (35.1731, -56.2792)
  arc A129 (34.2918, -56.2118) -> (35.1731, -56.2792) centre (34.7662, -55.8048) ccw
  arc A130 (34.8551, -58.7882) -> (33.9738, -58.7208) centre (34.3807, -59.1952) ccw
  line L145 (34.8551, -58.7882) -> (36.0482, -60.1791)
  line L146 (21.6569, -57.9744) -> (22.85, -59.3653)
  line L147 (20.7082, -58.7882) -> (21.9013, -60.1791)
  arc A131 (22.0446, -60.6812) -> (21.9013, -60.1791) centre (21.4269, -60.586) ccw
  arc A132 (22.85, -59.3653) -> (23.3244, -59.5833) centre (23.3244, -58.9583) ccw
  arc A133 (20.7082, -58.7882) -> (19.8269, -58.7208) centre (20.2338, -59.1952) ccw
  line L148 (19.8269, -58.7208) -> (18.0482, -60.2466)
  arc A134 (18.0482, -60.2466) -> (17.8374, -60.6258) centre (18.4551, -60.7209) ccw
  line L149 (17.8374, -60.6258) -> (16.6556, -68.301)
  line L150 (22.0446, -60.6812) -> (20.8628, -68.3563)
  line L151 (23.8098, -43.9923) -> (25.0029, -45.3831)
  arc A135 (24.1975, -46.699) -> (24.0542, -46.197) centre (23.5798, -46.6039) ccw
  line L152 (22.8611, -44.8061) -> (24.0542, -46.197)
  line L153 (21.9798, -44.7387) -> (20.2011, -46.2645)
  line L154 (24.1975, -46.699) -> (23.0157, -54.3742)
  arc A136 (20.2011, -46.2645) -> (19.9903, -46.6437) centre (20.608, -46.7388) ccw
  arc A137 (23.91, -55.4167) -> (23.5031, -55.5673) centre (23.91, -56.0417) ccw
  arc A138 (22.8049, -54.7534) -> (23.0157, -54.3742) centre (22.398, -54.2791) ccw
  line L155 (22.4541, -44.3317) -> (20.5519, -56.6861) construction
  line L156 (19.9903, -46.6437) -> (18.8085, -54.3188)
  arc A139 (21.7244, -57.0931) -> (21.6569, -57.9744) centre (22.1313, -57.5675) ccw
  line L157 (22.8049, -54.7534) -> (21.0262, -56.2792)
  line L158 (23.5031, -55.5673) -> (21.7244, -57.0931)
  arc A140 (20.1449, -56.2118) -> (21.0262, -56.2792) centre (20.6193, -55.8048) ccw
  arc A141 (32.15, -55.6347) -> (31.6756, -55.4167) centre (31.6756, -56.0417) ccw
  arc A142 (32.9554, -54.3188) -> (33.0987, -54.8209) centre (33.5731, -54.414) ccw
  line L159 (34.2918, -56.2118) -> (33.0987, -54.8209)
  line L160 (32.15, -55.6347) -> (33.3431, -57.0256)
  line L161 (31.4969, -59.4327) -> (33.2756, -57.9069)
  arc A143 (33.2756, -57.9069) -> (33.3431, -57.0256) centre (32.8687, -57.4325) ccw
  arc A144 (18.8085, -54.3188) -> (18.9518, -54.8209) centre (19.4262, -54.414) ccw
  line L162 (20.1449, -56.2118) -> (18.9518, -54.8209)
  arc A145 (30.8025, -68.301) -> (30.9458, -68.803) centre (31.4202, -68.3961) ccw
  arc A146 (31.09, -59.5833) -> (31.4969, -59.4327) centre (31.09, -58.9583) ccw
  line L163 (31.9843, -60.6258) -> (30.8025, -68.301)
  arc A147 (32.1951, -60.2466) -> (31.9843, -60.6258) centre (32.602, -60.7209) ccw
  line L164 (32.1389, -70.1939) -> (30.9458, -68.803)
  line L165 (34.7989, -68.7355) -> (33.0202, -70.2613)
  line L166 (36.1915, -60.6812) -> (35.0097, -68.3563)
  line L167 (33.9738, -58.7208) -> (32.1951, -60.2466)
  arc A148 (36.1915, -60.6812) -> (36.0482, -60.1791) centre (35.5738, -60.586) ccw
  arc A149 (38.3444, -46.699) -> (38.2011, -46.197) centre (37.7267, -46.6039) ccw
  arc A150 (34.3029, -41.6526) -> (33.8285, -41.4346) centre (33.8285, -42.0596) ccw
  line L168 (34.3029, -41.6526) -> (35.496, -43.0435)
  arc A151 (35.4285, -43.9248) -> (35.496, -43.0435) centre (35.0216, -43.4504) ccw
  line L169 (33.6498, -45.4506) -> (35.4285, -43.9248)
  arc A152 (37.008, -44.8061) -> (36.1266, -44.7387) centre (36.5336, -45.213) ccw
  line L170 (37.008, -44.8061) -> (38.2011, -46.197)
  arc A153 (33.2429, -45.6012) -> (33.6498, -45.4506) centre (33.2429, -44.9762) ccw
  arc A154 (21.7571, -69.3988) -> (21.3502, -69.5494) centre (21.7571, -70.0238) ccw
  line L171 (21.7571, -69.3988) -> (29.5227, -69.3988)
  arc A155 (28.9371, -73.5654) -> (29.344, -73.4148) centre (28.9371, -72.9404) ccw
  arc A156 (29.9971, -69.6169) -> (29.5227, -69.3988) centre (29.5227, -70.0238) ccw
  line L172 (29.344, -73.4148) -> (31.1227, -71.889)
  line L173 (29.9971, -69.6169) -> (31.1902, -71.0077)
  arc A157 (31.1227, -71.889) -> (31.1902, -71.0077) centre (30.7158, -71.4147) ccw
  arc A158 (32.1389, -70.1939) -> (33.0202, -70.2613) centre (32.6133, -69.787) ccw
  line L174 (21.1715, -73.5654) -> (28.9371, -73.5654)
  arc A159 (19.5715, -71.0752) -> (19.504, -71.9565) centre (19.9784, -71.5496) ccw
  line L175 (19.504, -71.9565) -> (20.6971, -73.3474)
  arc A160 (34.7989, -68.7355) -> (35.0097, -68.3563) centre (34.392, -68.2612) ccw
  arc A161 (20.6971, -73.3474) -> (21.1715, -73.5654) centre (21.1715, -72.9404) ccw
  arc A162 (20.6521, -68.7355) -> (20.8628, -68.3563) centre (20.2451, -68.2612) ccw
  line L176 (21.3502, -69.5494) -> (19.5715, -71.0752)
  line L177 (20.6521, -68.7355) -> (18.8734, -70.2613)
  arc A163 (17.992, -70.1939) -> (18.8734, -70.2613) centre (18.4664, -69.787) ccw
  line L178 (17.992, -70.1939) -> (16.7989, -68.803)
  arc A164 (16.6556, -68.301) -> (16.7989, -68.803) centre (17.2733, -68.3961) ccw
  line L179 (35.9029, -43.5179) -> (23.4029, -43.5179) construction
  line L180 (26.0629, -41.4346) -> (33.8285, -41.4346)
  arc A165 (26.0629, -41.4346) -> (25.656, -41.5852) centre (26.0629, -42.0596) ccw
  line L181 (25.656, -41.5852) -> (23.8773, -43.111)
  arc A166 (23.8773, -43.111) -> (23.8098, -43.9923) centre (24.2842, -43.5853) ccw
  arc A167 (22.8611, -44.8061) -> (21.9798, -44.7387) centre (22.3867, -45.213) ccw
  line L182 (27.5, -35) -> (27.5, -95) construction
  line L183 (43.915, -88.1494) -> (11.085, -88.1494) construction
  line L184 (11.085, -88.1494) -> (11.085, -76.0309) construction
  line L185 (11.085, -76.0309) -> (43.915, -76.0309) construction
  line L186 (43.915, -76.0309) -> (43.915, -88.1494) construction
  line L187 (27.5, -88.1494) -> (27.5, -76.0309) construction
  line L188 (55.5837, -83.5779) -> (56.7159, -83.5779)
  spline S0 degree 2 poles (56.7159, -83.5779) (56.7159, -84.0121) (57.1501, -84.3739) (57.563, -84.3739) knots 0 0 0 1 2 2 2
  spline S1 degree 2 poles (57.563, -84.3739) (57.9546, -84.3739) (58.4357, -83.9695) (58.4357, -83.6588) knots 0 0 0 1 2 2 2
  spline S2 degree 2 poles (58.4357, -83.6588) (58.4357, -83.2288) (57.8269, -82.9351) knots 0 0 0 1 1 1
  line L189 (57.8269, -82.9351) -> (57.0863, -82.5818)
  spline S3 degree 2 poles (57.0863, -82.5818) (56.252, -82.1817) (55.5198, -81.275) (55.5198, -80.6237) knots 0 0 0 1 2 2 2
  spline S4 degree 2 poles (55.5198, -80.6237) (55.5198, -79.815) (56.7202, -78.7636) (57.6269, -78.7636) knots 0 0 0 1 2 2 2
  spline S5 degree 2 poles (57.6269, -78.7636) (58.4995, -78.7636) (59.7169, -79.7554) (59.7169, -80.4833) knots 0 0 0 1 2 2 2
  spline S6 degree 2 poles (59.7169, -80.4833) (59.7169, -80.5429) (59.6999, -80.7642) knots 0 0 0 1 1 1
  line L190 (59.6999, -80.7642) -> (58.6059, -80.7642)
  spline S7 degree 2 poles (58.6059, -80.7642) (58.5719, -80.2704) (58.0568, -79.8065) (57.6354, -79.8065) knots 0 0 0 1 2 2 2
  spline S8 degree 2 poles (57.6354, -79.8065) (57.214, -79.8065) (56.6478, -80.2832) (56.6478, -80.6237) knots 0 0 0 1 2 2 2
  spline S9 degree 2 poles (56.6478, -80.6237) (56.6478, -80.9472) (57.2225, -81.4666) (57.9972, -81.8071) knots 0 0 0 1 2 2 2
  spline S10 degree 2 poles (57.9972, -81.8071) (58.8571, -82.186) (59.5637, -82.9862) (59.5637, -83.5949) knots 0 0 0 1 2 2 2
  spline S11 degree 2 poles (59.5637, -83.5949) (59.5637, -84.3952) (58.4016, -85.4168) (57.4949, -85.4168) knots 0 0 0 1 2 2 2
  spline S12 degree 2 poles (57.4949, -85.4168) (56.7287, -85.4168) (55.5837, -84.4718) (55.5837, -83.8205) knots 0 0 0 1 2 2 2
  line L191 (55.5837, -83.8205) -> (55.5837, -83.5779)
  line L192 (53.8171, -85.3402) -> (52.6934, -85.3402)
  line L193 (52.6934, -85.3402) -> (52.6934, -81.0409)
  spline S13 degree 2 poles (52.6934, -81.0409) (52.6934, -80.3811) (52.1613, -79.8065) (51.5696, -79.8065) knots 0 0 0 1 2 2 2
  spline S14 degree 2 poles (51.5696, -79.8065) (51.0119, -79.8065) (50.697, -80.1555) knots 0 0 0 1 1 1
  spline S15 degree 2 poles (50.697, -80.1555) (50.5607, -80.313) (50.4799, -80.645) (50.4799, -81.092) knots 0 0 0 1 2 2 2
  line L194 (50.4799, -81.092) -> (50.4799, -85.3402)
  line L195 (50.4799, -85.3402) -> (49.3561, -85.3402)
  line L196 (49.3561, -85.3402) -> (49.3561, -81.092)
  spline S16 degree 2 poles (49.3561, -81.092) (49.3561, -80.4535) (49.5604, -79.7256) (49.8286, -79.4191) knots 0 0 0 1 2 2 2
  spline S17 degree 2 poles (49.8286, -79.4191) (50.4075, -78.7636) (51.6164, -78.7636) knots 0 0 0 1 1 1
  spline S18 degree 2 poles (51.6164, -78.7636) (52.6678, -78.7636) (53.1063, -79.351) knots 0 0 0 1 1 1
  spline S19 degree 2 poles (53.1063, -79.351) (53.5745, -79.683) (53.8171, -80.4024) (53.8171, -80.9728) knots 0 0 0 1 2 2 2
  line L197 (53.8171, -80.9728) -> (53.8171, -85.3402)
  line L198 (43.5201, -83.5779) -> (44.6524, -83.5779)
  spline S20 degree 2 poles (44.6524, -83.5779) (44.6524, -84.0121) (45.0866, -84.3739) (45.4995, -84.3739) knots 0 0 0 1 2 2 2
  spline S21 degree 2 poles (45.4995, -84.3739) (45.8911, -84.3739) (46.3721, -83.9695) (46.3721, -83.6588) knots 0 0 0 1 2 2 2
  spline S22 degree 2 poles (46.3721, -83.6588) (46.3721, -83.2288) (45.7634, -82.9351) knots 0 0 0 1 1 1
  line L199 (45.7634, -82.9351) -> (45.0228, -82.5818)
  spline S23 degree 2 poles (45.0228, -82.5818) (44.1884, -82.1817) (43.4563, -81.275) (43.4563, -80.6237) knots 0 0 0 1 2 2 2
  spline S24 degree 2 poles (43.4563, -80.6237) (43.4563, -79.815) (44.6567, -78.7636) (45.5634, -78.7636) knots 0 0 0 1 2 2 2
  spline S25 degree 2 poles (45.5634, -78.7636) (46.436, -78.7636) (47.6534, -79.7554) (47.6534, -80.4833) knots 0 0 0 1 2 2 2
  spline S26 degree 2 poles (47.6534, -80.4833) (47.6534, -80.5429) (47.6364, -80.7642) knots 0 0 0 1 1 1
  line L200 (47.6364, -80.7642) -> (46.5424, -80.7642)
  spline S27 degree 2 poles (46.5424, -80.7642) (46.5083, -80.2704) (45.9933, -79.8065) (45.5719, -79.8065) knots 0 0 0 1 2 2 2
  spline S28 degree 2 poles (45.5719, -79.8065) (45.1505, -79.8065) (44.5843, -80.2832) (44.5843, -80.6237) knots 0 0 0 1 2 2 2
  spline S29 degree 2 poles (44.5843, -80.6237) (44.5843, -80.9472) (45.159, -81.4666) (45.9337, -81.8071) knots 0 0 0 1 2 2 2
  spline S30 degree 2 poles (45.9337, -81.8071) (46.7935, -82.186) (47.5002, -82.9862) (47.5002, -83.5949) knots 0 0 0 1 2 2 2
  spline S31 degree 2 poles (47.5002, -83.5949) (47.5002, -84.3952) (46.3381, -85.4168) (45.4314, -85.4168) knots 0 0 0 1 2 2 2
  spline S32 degree 2 poles (45.4314, -85.4168) (44.6652, -85.4168) (43.5201, -84.4718) (43.5201, -83.8205) knots 0 0 0 1 2 2 2
  line L201 (43.5201, -83.8205) -> (43.5201, -83.5779)
  line L202 (38.9697, -84.2973) -> (38.9697, -78.8402)
  line L203 (38.9697, -78.8402) -> (40.0935, -78.8402)
  line L204 (40.0935, -78.8402) -> (40.0935, -84.2973)
  line L205 (40.0935, -84.2973) -> (41.8004, -84.2973)
  line L206 (41.8004, -84.2973) -> (41.8004, -85.3402)
  line L207 (41.8004, -85.3402) -> (37.2372, -85.3402)
  line L208 (37.2372, -85.3402) -> (37.2372, -84.2973)
  line L209 (37.2372, -84.2973) -> (38.9697, -84.2973)
  line L210 (32.7081, -80.6621) -> (34.3342, -80.6621)
  line L211 (34.3342, -80.6621) -> (34.7939, -78.8402)
  line L212 (34.7939, -78.8402) -> (35.9262, -78.8402)
  line L213 (35.9262, -78.8402) -> (34.1809, -85.3402)
  line L214 (34.1809, -85.3402) -> (32.6953, -85.3402)
  line L215 (32.6953, -85.3402) -> (31.065, -78.8402)
  line L216 (31.065, -78.8402) -> (32.2739, -78.8402)
  line L217 (32.2739, -78.8402) -> (32.7081, -80.6621)
  line L218 (32.9294, -81.7049) -> (33.4913, -84.3271)
  line L219 (33.4913, -84.3271) -> (34.1, -81.7049)
  line L220 (34.1, -81.7049) -> (32.9294, -81.7049)
  line L221 (26.9062, -84.2973) -> (26.9062, -79.8831)
  line L222 (26.9062, -79.8831) -> (25.7526, -79.8831)
  line L223 (25.7526, -79.8831) -> (25.7526, -78.8402)
  line L224 (25.7526, -78.8402) -> (29.1708, -78.8402)
  line L225 (29.1708, -78.8402) -> (29.1708, -79.8831)
  line L226 (29.1708, -79.8831) -> (28.03, -79.8831)
  line L227 (28.03, -79.8831) -> (28.03, -84.2973)
  line L228 (28.03, -84.2973) -> (28.9835, -84.2973)
  line L229 (28.9835, -84.2973) -> (28.9835, -85.3402)
  line L230 (28.9835, -85.3402) -> (25.9527, -85.3402)
  line L231 (25.9527, -85.3402) -> (25.9527, -84.2973)
  line L232 (25.9527, -84.2973) -> (26.9062, -84.2973)
  line L233 (20.2827, -80.7174) -> (20.2827, -85.3402)
  line L234 (20.2827, -85.3402) -> (19.2356, -85.3402)
  line L235 (19.2356, -85.3402) -> (19.2356, -78.8402)
  line L236 (19.2356, -78.8402) -> (20.4232, -78.8402)
  line L237 (20.4232, -78.8402) -> (22.5729, -83.6758)
  line L238 (22.5729, -83.6758) -> (22.5729, -78.8402)
  line L239 (22.5729, -78.8402) -> (23.62, -78.8402)
  line L240 (23.62, -78.8402) -> (23.62, -85.3402)
  line L241 (23.62, -85.3402) -> (22.3472, -85.3402)
  line L242 (22.3472, -85.3402) -> (20.2827, -80.7174)
  line L243 (14.6128, -80.6621) -> (16.2389, -80.6621)
  line L244 (16.2389, -80.6621) -> (16.6986, -78.8402)
  line L245 (16.6986, -78.8402) -> (17.8309, -78.8402)
  line L246 (17.8309, -78.8402) -> (16.0856, -85.3402)
  line L247 (16.0856, -85.3402) -> (14.6, -85.3402)
  line L248 (14.6, -85.3402) -> (12.9697, -78.8402)
  line L249 (12.9697, -78.8402) -> (14.1786, -78.8402)
  line L250 (14.1786, -78.8402) -> (14.6128, -80.6621)
  line L251 (14.8342, -81.7049) -> (15.396, -84.3271)
  line L252 (15.396, -84.3271) -> (16.0047, -81.7049)
  line L253 (16.0047, -81.7049) -> (14.8342, -81.7049)
  line L254 (10.5434, -81.9476) -> (8.1852, -81.9476)
  line L255 (8.1852, -81.9476) -> (8.1852, -80.6791)
  line L256 (8.1852, -80.6791) -> (10.5434, -80.6791)
  line L257 (10.5434, -80.6791) -> (10.5434, -81.9476)
  spline S33 degree 2 poles (3.3197, -85.4168) (2.3237, -85.4168) (0.9956, -83.497) (0.9956, -82.1093) knots 0 0 0 1 2 2 2
  spline S34 degree 2 poles (0.9956, -82.1093) (0.9956, -80.6365) (2.2896, -78.7636) (3.3368, -78.7636) knots 0 0 0 1 2 2 2
  spline S35 degree 2 poles (3.3368, -78.7636) (4.3584, -78.7636) (5.6609, -80.6237) (5.6609, -82.0412) knots 0 0 0 1 2 2 2
  spline S36 degree 2 poles (5.6609, -82.0412) (5.6609, -83.48) (4.3414, -85.4168) (3.3197, -85.4168) knots 0 0 0 1 2 2 2
  spline S37 degree 2 poles (3.3197, -84.3739) (3.8731, -84.3739) (4.3456, -83.8333) knots 0 0 0 1 1 1
  spline S38 degree 2 poles (4.3456, -83.8333) (4.5329, -83.2246) (4.5329, -82.0497) knots 0 0 0 1 1 1
  spline S39 degree 2 poles (4.5329, -82.0497) (4.5329, -80.9643) (3.8901, -79.8065) (3.3325, -79.8065) knots 0 0 0 1 2 2 2
  spline S40 degree 2 poles (3.3325, -79.8065) (2.7791, -79.8065) (2.1236, -81.0026) (2.1236, -82.1136) knots 0 0 0 1 2 2 2
  spline S41 degree 2 poles (2.1236, -82.1136) (2.1236, -83.1607) (2.7877, -84.3739) (3.3197, -84.3739) knots 0 0 0 1 2 2 2
  line L258 (-1.8309, -81.4495) -> (-1.8309, -78.8402)
  line L259 (-1.8309, -78.8402) -> (-0.7071, -78.8402)
  line L260 (-0.7071, -78.8402) -> (-0.7071, -85.3402)
  line L261 (-0.7071, -85.3402) -> (-3.0398, -85.3402)
  spline S42 degree 2 poles (-3.0398, -85.3402) (-3.6144, -85.3402) (-4.3083, -85.0975) (-4.6616, -84.608) knots 0 0 0 1 2 2 2
  spline S43 degree 2 poles (-4.6616, -84.608) (-5.1852, -84.2334) (-5.1852, -83.3736) knots 0 0 0 1 1 1
  spline S44 degree 2 poles (-5.1852, -83.3736) (-5.1852, -82.518) (-4.5594, -81.9561) knots 0 0 0 1 1 1
  spline S45 degree 2 poles (-4.5594, -81.9561) (-3.9933, -81.4495) (-2.9717, -81.4495) knots 0 0 0 1 1 1
  line L262 (-2.9717, -81.4495) -> (-1.8309, -81.4495)
  line L263 (-1.8309, -82.4924) -> (-2.993, -82.4924)
  spline S46 degree 2 poles (-2.993, -82.4924) (-3.508, -82.4924) (-4.0571, -82.9607) (-4.0571, -83.3821) knots 0 0 0 1 2 2 2
  spline S47 degree 2 poles (-4.0571, -83.3821) (-4.0571, -84.2973) (-3.0015, -84.2973) knots 0 0 0 1 1 1
  line L264 (-3.0015, -84.2973) -> (-1.8309, -84.2973)
  line L265 (-1.8309, -84.2973) -> (-1.8309, -82.4924)
  point P0 (0, 0)
  point P1 (27.5, -57.5)
  point P2 (31.9629, -55.4167)
  point P3 (23.6787, -55.4167)
  point P4 (32.9117, -54.6028)
  point P5 (27.5, -57.5)
  point P6 (31.3213, -59.5833)
  point P7 (23.0371, -59.5833)
  point P8 (21.25, -57.5)
  point P9 (20.3012, -58.3139)
  point P10 (22.0883, -60.3972)
  point P11 (37.1274, -54.6028)
  point P12 (34.6988, -56.6861)
  point P13 (33.75, -57.5)
  point P14 (38.3881, -46.4151)
  point P15 (34.4481, -58.3139)
  point P16 (36.2352, -60.3972)
  point P17 (22.9805, -54.6028)
  point P18 (18.7648, -54.6028)
  point P19 (20.0255, -46.4151)
  point P20 (24.2412, -46.4151)
  point P21 (34.1724, -46.4151)
  point P22 (33.4742, -45.6012)
  point P23 (25.19, -45.6012)
  point P24 (36.601, -44.3317)
  point P25 (25.8316, -41.4346)
  point P26 (34.1158, -41.4346)
  point P27 (16.6119, -68.5849)
  point P28 (17.8726, -60.3972)
  point P29 (20.8276, -68.5849)
  point P30 (32.0195, -60.3972)
  point P31 (29.81, -69.3988)
  point P32 (21.5258, -69.3988)
  point P33 (30.7588, -68.5849)
  point P34 (32.5459, -70.6683)
  point P35 (19.0971, -71.4821)
  point P36 (20.8842, -73.5654)
  point P37 (29.1684, -73.5654)
  point P38 (18.399, -70.6683)
  point P39 (31.5971, -71.4821)
  point P40 (34.9745, -68.5849)
  point P41 (-17.2503, 20.1391)
  point P42 (3.6787, -55.4167)
  point P43 (7.5, -57.5)
  point P44 (11.9629, -55.4167)
  point P45 (11.3213, -59.5833)
  point P46 (3.0371, -59.5833)
  point P47 (12.9117, -54.6028)
  point P48 (5.19, -45.6012)
  point P49 (14.1724, -46.4151)
  point P50 (18.3881, -46.4151)
  point P51 (17.1274, -54.6028)
  point P52 (13.4742, -45.6012)
  point P53 (16.601, -44.3317)
  point P54 (7.5, -57.5)
  point P55 (14.6988, -56.6861)
  point P56 (13.75, -57.5)
  point P57 (14.4481, -58.3139)
  point P58 (16.2352, -60.3972)
  point P59 (1.25, -57.5)